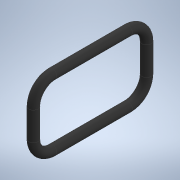
# Autodesk Inventor part: discharge_sealant
Saved by Autodesk Inventor 2020.2 (Build 242310000, 310)
## iProperties
Created: 2020-03-22
Part Number: discharge_sealant
Material: Rubber, Silicone
Document SubType Name: Modeling
Designer: agmle
Density: 1.25 g/cm^3
Appearance: Rubber - Black
Author: agmle
Autodesk Inventor part; units mm, degrees
ref_plane "YZ Plane" through (0, 0, 0) normal (1, 0, 0) x (0, 1, 0)
ref_plane "XZ Plane" through (0, 0, 0) normal (0, 1, 0) x (-1, 0, 0)
sketch "Sketch1" plane through (0, 0, 0) normal (1, 0, 0) x (0, 1, 0)
  line L0 (2, 0) -> (8, 0) construction
  line L1 (10, -2) -> (10, -18) construction
  line L2 (8, -20) -> (2, -20) construction
  line L3 (0, -18) -> (0, -2) construction
  arc A0 (10, -2) -> (8, 0) centre (8, -2) ccw construction
  arc A1 (8, -20) -> (10, -18) centre (8, -18) ccw construction
  arc A2 (0, -18) -> (2, -20) centre (2, -18) ccw construction
  arc A3 (2, 0) -> (0, -2) centre (2, -2) ccw construction
  line L4 (12, -18) -> (12, -2)
  arc A4 (12, -2) -> (8, 2) centre (8, -2) ccw
  line L5 (8, 2) -> (2, 2)
  arc A5 (2, 2) -> (-2, -2) centre (2, -2) ccw
  line L6 (-2, -2) -> (-2, -18)
  arc A6 (-2, -18) -> (2, -22) centre (2, -18) ccw
  line L7 (2, -22) -> (8, -22)
  arc A7 (8, -22) -> (12, -18) centre (8, -18) ccw
  point P0 (0, 0)
  dimension "d0" = 2
  dimension "d1" = 20
  dimension "d2" = 10
  dimension "d3" = 2
  constraints: 16 end point, 16 point on circle, 8 centre point, 8 tangent, 4 parallel, 3 equal radius, 2 perpendicular, 2 point on line, 1 horizontal, 7 other
  measures "d0" radius of A0
  measures "d1" distance between parallel lines of L2 L0
  measures "d2" distance between parallel lines of L3 L1
  measures "d3" distance between parallel lines of L1 L4
ref_plane "Work Plane1" through (0, 12, -2) normal (0, 0, 1) x (1, 0, 0)
sketch "Sketch2" plane through (0, 12, -2) normal (0, 0, 1) x (1, 0, 0)
  circle A0 centre (0, 0) radius 1
  point P0 (0, -12)
  dimension "d4" = 2
  constraints: 1 centre point
  measures "d4" diameter of A0
sweep "Sweep1" add profiles "Sketch2" path "Sketch1" path curves L4 A7 L7 A6 L6 A5 L5 A4
equation "\"d0\" = discharge_radius"
equation "\"d1\" = discharge_width"
equation "\"d2\" = discharge_height"
equation "\"discharge_radius\" = 2"
equation "\"discharge_width\" = 20"
equation "\"discharge_height\" = 10"
body "Solid1"
